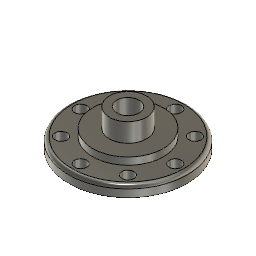
QWEQ (2) (Autodesk Fusion 360 design; units mm, degrees)
Autodesk Fusion 360 part; units mm, degrees
sketch "Sketch1" plane through (0, 0, 0) normal (0, 0, 1) x (1, 0, 0)
  circle A0 centre (50, 25) radius 2
extrude "Extrude1" add sketch "Sketch1" along normal blind 0.38
fillet "Fillet1" radius 0.12 1 edges at (48.1353, 24.2768, 0.38)
sketch "Sketch2" plane through (0, 0, 0.38) normal (0, 0, 1) x (-1, 0, 0)
  circle A0 centre (-50, -25) radius 1.88
  circle A1 centre (-50, -25) radius 1.19
  dimension "d4" = 2.38
  measures "d4" diameter of A1
extrude "Extrude2" add sketch "Sketch2" along normal blind 0.24 contours A1
sketch "Sketch3" plane through (0, 0, 0.62) normal (0, 0, 1) x (-1, 0, 0)
  circle A0 centre (-50, -25) radius 1.19
  circle A1 centre (-50, -25) radius 0.375
  dimension "d7" = 0.75
  measures "d7" diameter of A1
extrude "Extrude3" add sketch "Sketch3" along normal blind 0.63 contours A1
sketch "Sketch4" plane through (0, 0, 0) normal (0, 0, -1) x (1, 0, 0)
  circle A0 centre (50, -25) radius 2
  circle A1 centre (50, -25) radius 0.875
  dimension "d10" = 1.75
  measures "d10" diameter of A1
extrude "Extrude4" cut sketch "Sketch4" against normal blind 0.187 contours A1
sketch "Sketch5" plane through (0, 0, 0.62) normal (0, 0, 1) x (-1, 0, 0)
  circle A0 centre (-50, -25) radius 0.375
  circle A1 centre (-50, -25) radius 1.19
  circle A2 centre (-50, -25) radius 0.625
  dimension "d13" = 1.25
  measures "d13" diameter of A2
extrude "Extrude5" add sketch "Sketch5" along normal blind 0.63 contours A2
sketch "Sketch6" plane through (0, 0, 1.25) normal (0, 0, 1) x (-1, 0, 0)
  circle A0 centre (-50, -25) radius 0.625
  circle A1 centre (-50, -25) radius 0.375
  dimension "d16" = 0.75
  measures "d16" diameter of A1
extrude "Extrude6" cut sketch "Sketch6" against normal blind 1.063 contours A1
sketch "Sketch7" plane through (0, 0, 0) normal (0, 0, -1) x (1, 0, 0)
  circle A0 centre (50, -25) radius 0.875
  circle A1 centre (50, -25) radius 2
  line L0 (50, -25) -> (51.39, -25)
  circle A2 centre (51.595, -25) radius 0.205
  arc A3 (51.5818, -24.7954) -> (51.5818, -25.2046) centre (50, -25) ccw
  dimension "d19" = 3.19
  dimension "d20" = 1.595
  dimension "d21" = 0.41
  measures "d19" diameter of A3
  measures "d21" diameter of A2
extrude "Extrude7" cut sketch "Sketch7" against normal blind 0.38 contours A2
sketch "Sketch8" plane through (0, 0, 0) normal (0, 0, -1) x (1, 0, 0)
  circle A0 centre (51.595, -25) radius 0.205
  circle A1 centre (50, -25) radius 0.875
  circle A2 centre (50, -25) radius 2
  circle A3 centre (51.1278, -23.8722) radius 0.205
  dimension "d24" = 1.595
  dimension "d25" = 0.41
  measures "d25" diameter of A3
extrude "Extrude8" cut sketch "Sketch8" against normal blind 0.38 contours A3
sketch "Sketch9" plane through (0, 0, 0) normal (0, 0, -1) x (1, 0, 0)
  circle A0 centre (51.1278, -23.8722) radius 0.205
  circle A1 centre (51.595, -25) radius 0.205
  circle A2 centre (50, -25) radius 0.875
  circle A3 centre (50, -25) radius 2
  circle A4 centre (50, -23.405) radius 0.205
  dimension "d28" = 1.595
  dimension "d29" = 0.41
  measures "d29" diameter of A4
extrude "Extrude9" cut sketch "Sketch9" against normal blind 0.38 contours A4
sketch "Sketch10" plane through (0, 0, 0) normal (0, 0, -1) x (1, 0, 0)
  circle A0 centre (50, -23.405) radius 0.205
  circle A1 centre (51.1278, -23.8722) radius 0.205
  circle A2 centre (51.595, -25) radius 0.205
  circle A3 centre (50, -25) radius 0.875
  circle A4 centre (50, -25) radius 2
  line L0 (50, -25) -> (51.595, -25) construction
  circle A5 centre (48.8722, -23.8722) radius 0.205
  dimension "d33" = 1.595
  dimension "d34" = 0.41
  measures "d34" diameter of A5
extrude "Extrude10" cut sketch "Sketch10" against normal blind 0.38 contours A5
sketch "Sketch11" plane through (0, 0, 0) normal (0, 0, -1) x (1, 0, 0)
  circle A0 centre (48.8722, -23.8722) radius 0.205
  circle A1 centre (50, -23.405) radius 0.205
  circle A2 centre (51.1278, -23.8722) radius 0.205
  circle A3 centre (51.595, -25) radius 0.205
  circle A4 centre (50, -25) radius 0.875
  circle A5 centre (50, -25) radius 2
  circle A6 centre (48.405, -25) radius 0.205
  dimension "d37" = 1.595
  dimension "d38" = 0.41
  measures "d38" diameter of A6
extrude "Extrude11" cut sketch "Sketch11" against normal blind 0.38 contours A6
sketch "Sketch12" plane through (0, 0, 0) normal (0, 0, -1) x (1, 0, 0)
  circle A0 centre (48.405, -25) radius 0.205
  circle A1 centre (48.8722, -23.8722) radius 0.205
  circle A2 centre (50, -23.405) radius 0.205
  circle A3 centre (51.1278, -23.8722) radius 0.205
  circle A4 centre (51.595, -25) radius 0.205
  circle A5 centre (50, -25) radius 0.875
  circle A6 centre (50, -25) radius 2
  circle A7 centre (51.1278, -26.1278) radius 0.205
  dimension "d41" = 1.595
  dimension "d42" = 0.41
  measures "d42" diameter of A7
extrude "Extrude12" cut sketch "Sketch12" against normal blind 0.38 contours A7
sketch "Sketch13" plane through (0, 0, 0) normal (0, 0, -1) x (1, 0, 0)
  circle A0 centre (51.1278, -26.1278) radius 0.205
  circle A1 centre (48.405, -25) radius 0.205
  circle A2 centre (48.8722, -23.8722) radius 0.205
  circle A3 centre (50, -23.405) radius 0.205
  circle A4 centre (51.1278, -23.8722) radius 0.205
  circle A5 centre (51.595, -25) radius 0.205
  circle A6 centre (50, -25) radius 0.875
  circle A7 centre (50, -25) radius 2
  circle A8 centre (50, -26.595) radius 0.205
  dimension "d45" = 1.595
  dimension "d46" = 0.41
  measures "d46" diameter of A8
extrude "Extrude13" cut sketch "Sketch13" against normal blind 0.38 contours A8
sketch "Sketch14" plane through (0, 0, 0) normal (0, 0, -1) x (1, 0, 0)
  circle A0 centre (50, -26.595) radius 0.205
  circle A1 centre (51.1278, -26.1278) radius 0.205
  circle A2 centre (48.405, -25) radius 0.205
  circle A3 centre (48.8722, -23.8722) radius 0.205
  circle A4 centre (50, -23.405) radius 0.205
  circle A5 centre (51.1278, -23.8722) radius 0.205
  circle A6 centre (51.595, -25) radius 0.205
  circle A7 centre (50, -25) radius 0.875
  circle A8 centre (50, -25) radius 2
  line L0 (50, -25) -> (51.595, -25) construction
  circle A9 centre (48.8722, -26.1278) radius 0.205
  dimension "d50" = 1.595
  dimension "d51" = 0.41
  measures "d51" diameter of A9
extrude "Extrude14" cut sketch "Sketch14" against normal blind 0.38 contours A9
